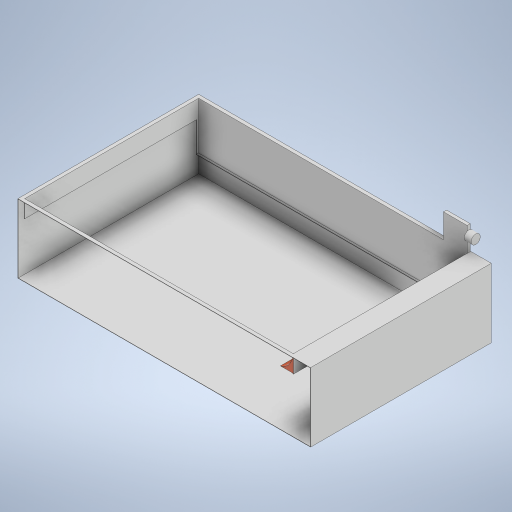
# Autodesk Inventor part: cubre
Saved by Autodesk Inventor 2023 (Build 270158000, 158)
## iProperties
Created: 2022-04-05
Part Number: cubre
Material: Genérico
Document SubType Name: Modeling
Designer: isaac
Density: 1 g/cm^3
Appearance: Valor por defecto
Author: isaac
Autodesk Inventor part; units mm, degrees
ref_plane "YZ Plane" through (0, 0, 0) normal (1, 0, 0) x (0, 1, 0)
ref_plane "XZ Plane" through (0, 0, 0) normal (0, 1, 0) x (-1, 0, 0)
ref_plane "XY Plane" through (0, 0, 0) normal (0, 0, 1) x (1, 0, 0)
sketch "Boceto1" plane through (0, 0, 0) normal (0, 0, 1) x (1, 0, 0)
  line L0 (-425, 100) -> (425, 100)
  line L1 (425, 100) -> (425, -100)
  line L2 (425, -100) -> (-425, -100)
  line L3 (-425, -100) -> (-425, 100)
  point P0 (0, 0)
  point P1 (425, 0)
  point P2 (0, 100)
  dimension "d0" = 200
  dimension "d1" = 850
  constraints: 8 end point, 2 midpoint, 2 parallel, 1 horizontal, 1 horizontal alignment, 1 perpendicular, 1 vertical alignment
  measures "d0" distance between parallel lines of L2 L0
  measures "d1" distance from line of point (425, 0) L3
extrude "Extrusión1" add sketch "Boceto1" along normal blind 525
sketch "Boceto2" plane through (-425, 100, 0) normal (0, 1, 0) x (1, 0, 0)
  line L0 (10, -515) -> (790, -515)
  line L1 (790, -515) -> (790, -10)
  line L2 (790, -10) -> (10, -10)
  line L3 (10, -10) -> (10, -515)
  line L4 (850, 0) -> (0, 0) construction
  line L5 (0, 0) -> (0, -525) construction
  line L6 (850, -525) -> (0, -525) construction
  line L7 (850, 0) -> (850, -525) construction
  point P0 (425, 0)
  dimension "d4" = 10
  dimension "d5" = 10
  dimension "d6" = 10
  dimension "d7" = 60
  constraints: 8 end point, 2 parallel, 1 horizontal, 1 perpendicular
  measures "d4" distance between parallel lines of L4 L2
  measures "d5" distance between parallel lines of L6 L0
  measures "d6" distance between parallel lines of L5 L3
  measures "d7" distance between parallel lines of L1 L7
extrude "Extrusión2" cut sketch "Boceto2" against normal blind 138
shell "Vaciado1" thickness 1 removed faces 1 at (-141.6667, 33.3333, 525)
shell "Vaciado2" thickness 1 removed faces 2 at (-155.3333, 53, 516) at (-155, 54, 515)
sketch "Boceto3" plane through (-425, 100, 0) normal (0, 1, 0) x (1, 0, 0)
  line L0 (10, -10) -> (790, -10) construction
  line L1 (790, -10) -> (790, -515) construction
  line L2 (790, -515) -> (10, -515) construction
  line L3 (10, -515) -> (10, -10) construction
  line L4 (850, 0) -> (0, 0) construction
  line L5 (0, 0) -> (0, -525) construction
  line L6 (850, -525) -> (0, -525) construction
  line L7 (850, 0) -> (850, -525) construction
  line L8 (849, -1) -> (1, -1) projected
  line L9 (721.1252, -10) -> (790, -10)
  line L10 (790, -10) -> (790, -1)
  line L11 (790, -1) -> (721.1252, -1)
  line L12 (721.1252, -1) -> (721.1252, -10)
  point P0 (425, 0)
  point P1 (790, -5.5)
  point P2 (721.1252, -5.5)
  point P3 (721.1252, -1)
  dimension "d12" = 68.8748
  constraints: 8 end point, 2 midpoint, 2 parallel, 2 point on line, 1 horizontal, 1 perpendicular, 1 vertical alignment
  measures "d12" distance of point (790, -5.5) point (721.125, -5.5)
extrude "Extrusión3" add sketch "Boceto3" along normal blind 70
sketch "Boceto4" plane through (365, 100, 10) normal (1, 0, 0) x (0, 0, -1)
  circle A0 centre (4.62, 43) radius 13.5
  line L0 (10, 0) -> (-515, 0) projected
  line L1 (9, 0) -> (9, 70) construction
  point P0 (10, -100)
  dimension "d15" = 27
  dimension "d16" = 43
  dimension "d17" = 4.38
  constraints: 1 centre point
  measures "d15" diameter of A0
  measures "d16" distance from line of L0 A0.centre
  measures "d17" distance from line of L1 A0.centre
extrude "Extrusión4" add sketch "Boceto4" along normal blind 20
sketch "Boceto5" plane through (-416, -39, 516) normal (0, 0, 1) x (1, 0, 0)
  line L0 (1, 139) -> (712.1252, 139) construction
  line L1 (1, 139) -> (1, 1) construction
  line L2 (1, 1) -> (781, 1) construction
  line L3 (781, 139) -> (781, 1) construction
  line L4 (781, 139) -> (781, 169.3151) construction
  line L5 (781, 169.3151) -> (781, 194.6849) construction
  line L6 (781, 194.6849) -> (781, 209) construction
  line L7 (712.1252, 209) -> (781, 209) construction
  line L8 (712.1252, 139) -> (712.1252, 209) construction
  line L9 (-8, -60) -> (840, -60) construction
  line L10 (840, -60) -> (840, 138) construction
  line L11 (840, 138) -> (-8, 138) construction
  line L12 (-8, 138) -> (-8, -60) construction
  line L13 (782, 138) -> (782, 0) construction
  line L14 (841, 139) -> (-9, 139) construction
  line L15 (-8, 138) -> (840, 138) construction
  line L16 (781, 138) -> (781, 1) projected
  line L17 (781, 90.481) -> (781, 138)
  arc A0 (744.2128, 90.481) -> (781, 138) centre (731.9157, 138) ccw
  line L18 (744.2128, 90.481) -> (781, 90.481)
  point P0 (416, 39)
  point P1 (716.6309, 139)
  constraints: 4 end point, 2 point on circle, 1 centre point, 1 collinear, 1 perpendicular, 1 point on line, 1 tangent
extrude "Extrusión5" add sketch "Boceto5" against normal through all
sketch "Boceto6" plane through (-416, -39, 516) normal (0, 0, 1) x (1, 0, 0)
  line L0 (784.0971, 88.443) -> (-3.152, 88.443)
  line L1 (-3.152, 88.443) -> (-3.152, -16.5059)
  line L2 (-3.152, -16.5059) -> (784.0971, -16.5059)
  line L3 (784.0971, -16.5059) -> (784.0971, 88.443)
  point P0 (416, 39)
  constraints: 8 end point, 2 parallel, 1 horizontal, 1 perpendicular
extrude "Extrusión6" cut sketch "Boceto6" against normal blind 500
